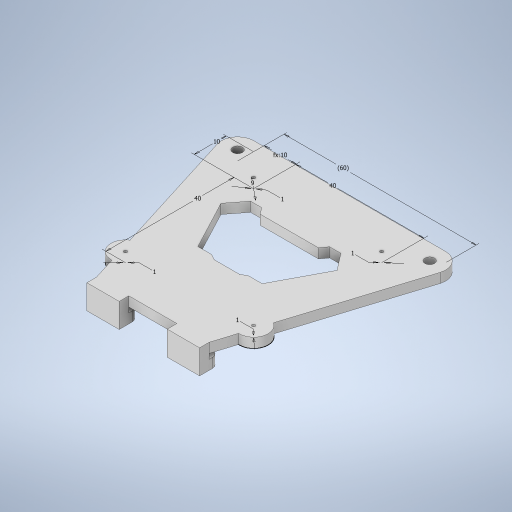
# Autodesk Inventor part: ElectronicsMount - ClipOnStyle
Saved by Autodesk Inventor 2023 (Build 270158000, 158)
## iProperties
Created: 2022-12-06
Part Number: ElectronicsMount - ClipOnStyle
Material: Generic
Document SubType Name: Modeling
Designer: Administrator
Density: 1 g/cm^3
Appearance: Default
Author: Administrator
Autodesk Inventor part; units mm, degrees
ref_plane "YZ Plane" through (0, 0, 0) normal (1, 0, 0) x (0, 1, 0)
ref_plane "XZ Plane" through (0, 0, 0) normal (0, 1, 0) x (-1, 0, 0)
sketch "Sketch1" plane through (0, 0, 0) normal (0, 1, 0) x (-1, 0, 0)
  line L0 (12.4, 56.4645) -> (22.5, 56.4645) construction
  circle A0 centre (0, 0) radius 1.5
  line L1 (12.4, 56.4645) -> (0, 0) construction
  circle A1 centre (60, 0) radius 1.5
  line L2 (0, 0) -> (60, 0) construction
  line L3 (47.6, 56.4645) -> (37.5, 56.4645) construction
  line L4 (60, 0) -> (47.6, 56.4645) construction
  line L5 (47.6, 56.4645) -> (37.5, 56.4645) construction
  line L6 (36, 58.4645) -> (24, 58.4645) construction
  line L7 (37.5, 56.4645) -> (36, 58.4645) construction
  line L8 (36, 58.4645) -> (24, 58.4645) construction
  line L9 (24, 58.4645) -> (22.5, 56.4645) construction
  line L10 (22.5, 56.4645) -> (12.4, 56.4645) construction
  line L11 (47.6, 56.4645) -> (47.6, 59.4645)
  line L12 (47.6, 59.4645) -> (37.5, 59.4645)
  line L13 (37.5, 59.4645) -> (37.5, 56.4645)
  line L14 (37.5, 56.4645) -> (22.5, 56.4645)
  line L15 (22.5, 56.4645) -> (22.5, 59.4645)
  line L16 (22.5, 59.4645) -> (12.4, 59.4645)
  line L17 (12.4, 59.4645) -> (12.4, 56.4645)
  circle A2 centre (60, 0) radius 5
  circle A3 centre (0, 0) radius 5
  line L18 (47.6, 56.4645) -> (64.7726, 1.4908)
  line L19 (12.4, 56.4645) -> (-4.7726, 1.4908)
  line L20 (0, -5) -> (60, -5)
  point P0 (17, 90.5)
  dimension "d0" = 3
  dimension "d1" = 10.1
  dimension "d2" = 3
  dimension "d3" = 10.1
  dimension "d4" = 10
  dimension "d5" = 10
  dimension "d6" = 3
  dimension "d7" = 3
  constraints: 42 end point, 4 centre point, 4 perpendicular, 4 point on circle, 3 coincident, 2 collinear, 2 point on line, 2 tangent, 1 horizontal, 1 parallel
  measures "d0" distance of L3.start L11.end
  measures "d1" distance of L11.end L12.end
  measures "d2" distance of L14.end L15.end
  measures "d3" distance of L15.end L16.end
  measures "d4" diameter of A2
  measures "d5" diameter of A3
  measures "d6" diameter of A1
  measures "d7" diameter of A0
extrude "Extrusion1" add sketch "Sketch1" along normal blind 3
sketch "Sketch2" plane through (0, 3, 0) normal (0, 1, 0) x (1, 0, 0)
  line L0 (-47.6, -56.4645) -> (-47.6, -59.4645) projected
  line L1 (-37.5, -59.4645) -> (-37.5, -56.4645) projected
  line L2 (-47.6, -59.4645) -> (-37.5, -59.4645)
  line L3 (-37.5, -59.4645) -> (-37.5, -56.4645)
  line L4 (-37.5, -56.4645) -> (-47.6, -56.4645)
  line L5 (-47.6, -56.4645) -> (-47.6, -59.4645)
  line L6 (-12.4, -59.4645) -> (-12.4, -56.4645) projected
  line L7 (-37.5, -56.4645) -> (-22.5, -56.4645) projected
  line L8 (-12.4, -59.4645) -> (-22.5, -59.4645)
  line L9 (-22.5, -59.4645) -> (-22.5, -56.4645)
  line L10 (-22.5, -56.4645) -> (-12.4, -56.4645)
  line L11 (-12.4, -56.4645) -> (-12.4, -59.4645)
  point P0 (0, 0)
  constraints: 16 end point, 4 parallel, 2 horizontal, 2 perpendicular
extrude "Extrusion2" add sketch "Sketch2" along normal blind 4.6
ref_plane "Work Plane1" through (-12.4, 3, 56.4645) normal (0, 0, 1) x (0, 1, 0)
sketch "Sketch3" plane through (-12.4, 3, 56.4645) normal (0, 0, 1) x (0, 1, 0)
  line L0 (0, 0) -> (4.6, 0) projected
  line L1 (-3, 10.1) -> (4.6, 10.1) projected
  line L2 (4.6, 0) -> (1.6, 0)
  line L3 (1.6, 0) -> (1.6, 10.1)
  line L4 (1.6, 10.1) -> (4.6, 10.1)
  line L5 (4.6, 10.1) -> (4.6, 0)
  line L6 (-3, 25.1) -> (4.6, 25.1) projected
  line L7 (-3, 35.2) -> (4.6, 35.2) projected
  line L8 (4.6, 25.1) -> (1.6, 25.1)
  line L9 (1.6, 25.1) -> (1.6, 35.2)
  line L10 (1.6, 35.2) -> (4.6, 35.2)
  line L11 (4.6, 35.2) -> (4.6, 25.1)
  point P0 (-3, -12.4)
  point P1 (1.6, 25.1)
  dimension "d12" = 3
  dimension "d13" = 3
  constraints: 16 end point, 4 parallel, 2 horizontal, 2 perpendicular, 2 point on line
  measures "d12" distance of L3.end L4.end
  measures "d13" distance of L9.end L10.end
extrude "Extrusion3" add sketch "Sketch3" against normal blind 3
fillet "Fillet1" radius 2 4 edges at (-12.4, 6.1, 53.4645) (-22.5, 6.1, 53.4645) (-37.5, 6.1, 53.4645) (-47.6, 6.1, 53.4645)
sketch "Sketch4" plane through (0, 3, 0) normal (0, 1, 0) x (1, 0, 0)
  circle A0 centre (-10, -5) radius 4.5
  line L0 (0, 5) -> (-60, 5) projected
  circle A1 centre (0, 0) radius 1.5 construction
  line L1 (0, 0) -> (0, -9.5) construction
  circle A2 centre (-50, -5) radius 4.5
  circle A3 centre (-10, -45) radius 4.5
  circle A4 centre (-50, -45) radius 4.5
  circle A5 centre (-10, -5) radius 0.5
  circle A6 centre (-50, -5) radius 0.5
  circle A7 centre (-50, -45) radius 0.5
  circle A8 centre (-10, -45) radius 0.5
  dimension "d18" = 9
  dimension "d27" = 60
  dimension "d28" = 10
  dimension "d29" = 10
  dimension "d32" = 40
  dimension "d35" = 40
  dimension "d53" = 1
  dimension "d54" = 1
  dimension "d55" = 1
  dimension "d56" = 1
  constraints: 8 centre point, 4 coincident, 2 end point, 2 vertical, 1 horizontal, 6 other
  measures "d18" diameter of A0
  measures "d27" distance of L0.start L0.end
  measures "d28" horizontal distance of point (0, 0) A0.centre
  measures "d29" distance from line of L0 A0.centre
  measures "d32" distance of A0.centre A2.centre
  measures "d35" distance of A0.centre A3.centre
  measures "d53" diameter of A5
  measures "d54" diameter of A6
  measures "d55" diameter of A7
  measures "d56" diameter of A8
extrude "Extrusion4" add sketch "Sketch4" against normal blind 3 contours A0 | A2 | A3 | A4 | A5 | A6 | A7 | A8
sketch "Sketch6" plane through (0, 0, 0) normal (0, -1, 0) x (1, 0, 0)
  circle A0 centre (-60, 0) radius 1.55 construction
  line L0 (-44.1169, 11.8645) -> (-48.1306, 17.0674)
  line L1 (-60, 0) -> (-44.1169, 11.8645) construction
  line L2 (-44.1169, 11.8645) -> (-48.1306, 17.0674)
  line L3 (-48.1306, 17.0674) -> (-40.0449, 32.3645)
  line L4 (-48.1306, 17.0674) -> (-40.0449, 32.3645)
  line L5 (-40.0449, 32.3645) -> (-35.7189, 32.3645)
  line L6 (-40.0449, 32.3645) -> (-35.7189, 32.3645)
  line L7 (-33.9689, 33.3645) -> (-26.0311, 33.3645)
  line L8 (-35.7189, 32.3645) -> (-33.9689, 33.3645)
  line L9 (-33.9689, 33.3645) -> (-26.0311, 33.3645)
  line L10 (-24.2811, 32.3645) -> (-19.9551, 32.3645)
  line L11 (-26.0311, 33.3645) -> (-24.2811, 32.3645)
  line L12 (-24.2811, 32.3645) -> (-19.9551, 32.3645)
  line L13 (-19.9551, 32.3645) -> (-11.8694, 17.0674)
  line L14 (-11.8694, 17.0674) -> (-15.9122, 11.8645)
  line L15 (-15.8831, 11.8645) -> (-19.4, 11.8645)
  line L16 (-15.9122, 11.8645) -> (-19.4, 11.8645)
  line L17 (-19.4, 11.8645) -> (-20.9, 13.8645)
  line L18 (-19.4, 11.8645) -> (-20.9, 13.8645)
  line L19 (-20.9, 13.8645) -> (-39.1, 13.8645)
  line L20 (-20.9, 13.8645) -> (-39.1, 13.8645)
  line L21 (-39.1, 13.8645) -> (-40.6, 11.8645)
  line L22 (-39.1, 13.8645) -> (-40.6, 11.8645)
  line L23 (-40.6, 11.8645) -> (-44.1169, 11.8645)
  line L24 (-40.6, 11.8645) -> (-44.1169, 11.8645)
  circle A1 centre (-60, 0) radius 1.5 construction
  point P0 (0, 0)
  point P1 (17, 90.5)
  constraints: 50 end point, 10 collinear, 2 coincident, 1 centre point
extrude "Extrusion6" cut sketch "Sketch6" against normal up to next
extrude "Extrusion8" cut sketch "Sketch4" against normal up to next contours A5 | A6 | A7 | A8
equation "\"d28\" = -0.5 * d22 + 0.5 * d27"
equation "\"d22\" = 40"
body "Solid1"
